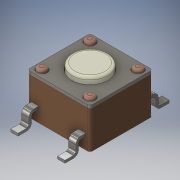
# Autodesk Inventor part: FSM2JSMAA
Saved by Autodesk Inventor 2016 (Build 200138000, 138)
## iProperties
Created: 2016-07-01
Part Number: FSM2JSMAA
Material: Generic
Document SubType Name: Modeling
Designer: Jonathan
Density: 1 g/cm^3
Appearance: Default
Author: Jonathan
Autodesk Inventor part; units mm, degrees
ref_plane "YZ Plane" through (0, 0, 0) normal (1, 0, 0) x (0, 1, 0)
ref_plane "XZ Plane" through (0, 0, 0) normal (0, 1, 0) x (-1, 0, 0)
ref_plane "XY Plane" through (0, 0, 0) normal (0, 0, 1) x (1, 0, 0)
sketch "Sketch1" plane through (0, 0, 0) normal (0, 1, 0) x (-1, 0, 0)
  line L0 (3, 3) -> (-3, 3)
  line L1 (-3, 3) -> (-3, -3)
  line L2 (-3, -3) -> (3, -3)
  line L3 (3, -3) -> (3, 3)
  point P0 (0, 0)
  point P1 (3, 0)
  point P2 (0, -3)
  dimension "d0" = 6
  dimension "d1" = 6
  constraints: 8 end point, 2 midpoint, 2 parallel, 1 horizontal, 1 horizontal alignment, 1 perpendicular, 1 vertical alignment
  measures "d0" distance of L2.end L0.start
  measures "d1" distance of L1.end L2.end
extrude "Extrusion1" add sketch "Sketch1" along normal blind 3.57
ref_plane "Work Plane1" through (2.25, 0, 3) normal (1, 0, 0) x (0, 0, -1)
sketch "Sketch2" plane through (2.25, 0, 3) normal (1, 0, 0) x (0, 0, -1)
  line L0 (6.45, 1.4) -> (6, 1.4)
  line L1 (6, 1.4) -> (6, 1.15)
  line L2 (6, 1.15) -> (6.45, 1.15)
  line L3 (6.7, 0.9) -> (6.7, 0.4)
  line L4 (6.95, 0.9) -> (6.95, 0.4)
  line L5 (7.2, 0.15) -> (8, 0.15)
  line L6 (8, 0.15) -> (8, -0.1)
  line L7 (8, -0.1) -> (7.2, -0.1)
  arc A0 (6.7, 0.9) -> (6.45, 1.15) centre (6.45, 0.9) ccw
  arc A1 (6.95, 0.9) -> (6.45, 1.4) centre (6.45, 0.9) ccw
  arc A2 (6.95, 0.4) -> (7.2, 0.15) centre (7.2, 0.4) ccw
  arc A3 (6.7, 0.4) -> (7.2, -0.1) centre (7.2, 0.4) ccw
  line L8 (6, 0) -> (6, 3.57) projected
  line L9 (0, 0) -> (6, 0) projected
  point P0 (3, 0)
  dimension "d6" = 0.25
  dimension "d7" = 0.8
  dimension "d8" = 2
  dimension "d9" = 1.5
  dimension "d11" = 0.1
  dimension "d12" = 0.7
  constraints: 16 end point, 8 point on circle, 8 tangent, 4 centre point, 4 perpendicular, 2 concentric, 2 horizontal, 2 vertical, 1 collinear, 1 equal radius
  measures "d6" distance between parallel lines of L3 L4
  measures "d7" distance of L6.end L7.end
  measures "d8" distance between parallel lines of L1 L6
  measures "d9" distance between parallel lines of L0 L7
  measures "d11" distance between parallel lines of L9 L7
  measures "d12" distance between parallel lines of L8 L3
extrude "Extrusion2" add sketch "Sketch2" along normal mid plane 0.7 separate body
mirror "Mirror1" about plane through (0, 0, 0) normal (1, 0, 0) of "Extrusion2" bodies 2
mirror "Mirror2" about plane through (0, 0, 0) normal (0, 0, 1) of "Extrusion2", "Mirror1" bodies 2
sketch "Sketch3" plane through (0, 3.57, 0) normal (0, 1, 0) x (1, 0, 0)
  line L0 (-3, -3) -> (3, -3) projected
  line L1 (3, 3) -> (-3, 3) projected
  line L2 (-3, -3) -> (3, -3)
  line L3 (3, -3) -> (3, 3)
  line L4 (3, 3) -> (-3, 3)
  line L5 (-3, 3) -> (-3, -3)
  circle A0 centre (0, 0) radius 1.75
  circle A1 centre (-2.3, -2.3) radius 0.5
  circle A2 centre (-2.3, 2.3) radius 0.5
  circle A3 centre (2.3, 2.3) radius 0.5
  circle A4 centre (2.3, -2.3) radius 0.5
  line L6 (-3, 3) -> (-3, -3) projected
  line L7 (-3, -3) -> (-2.3, -2.3) construction
  line L8 (-3, 3) -> (-2.3, 2.3) construction
  line L9 (2.3, 2.3) -> (3, 3) construction
  line L10 (3, -3) -> (3, 3) projected
  line L11 (2.3, -2.3) -> (3, -3) construction
  line L12 (-2.3, -2.3) -> (2.3, -2.3) construction
  line L13 (2.3, 2.3) -> (-2.3, 2.3) construction
  line L14 (-2.3, -2.3) -> (-2.3, 2.3) construction
  line L15 (2.3, 2.3) -> (2.3, -2.3) construction
  dimension "d15" = 3.5
  dimension "d16" = 1
  dimension "d17" = 0.7
  constraints: 24 end point, 5 centre point, 5 perpendicular, 4 parallel, 3 equal radius, 2 horizontal, 2 horizontal alignment, 2 vertical alignment, 1 coincident, 1 point on line
  measures "d15" diameter of A0
  measures "d16" diameter of A1
  measures "d17" distance from line of L5 L7.end
extrude "Extrusion3" add sketch "Sketch3" along normal blind 0.3 separate body
sketch "Sketch4" plane through (0, 3.57, 0) normal (0, 1, 0) x (1, 0, 0)
  circle A0 centre (-2.3, -2.3) radius 0.45
  circle A1 centre (-2.3, 2.3) radius 0.45
  circle A2 centre (2.3, 2.3) radius 0.45
  circle A3 centre (2.3, -2.3) radius 0.45
  circle A4 centre (-2.3, -2.3) radius 0.5 projected
  circle A5 centre (-2.3, 2.3) radius 0.5 projected
  circle A6 centre (2.3, 2.3) radius 0.5 projected
  circle A7 centre (2.3, -2.3) radius 0.5 projected
  point P0 (0, 0)
  dimension "d25" = 0.9
  dimension "d26" = 0.9
  dimension "d27" = 0.9
  dimension "d28" = 0.9
  constraints: 4 centre point, 4 concentric
  measures "d25" diameter of A0
  measures "d26" diameter of A3
  measures "d27" diameter of A2
  measures "d28" diameter of A1
extrude "Extrusion4" add sketch "Sketch4" along normal blind 0.6 separate body contours A0 | A1 | A2 | A3
sketch "Sketch5" plane through (0, 3.57, 0) normal (0, 1, 0) x (1, 0, 0)
  circle A0 centre (0, 0) radius 1.7
  circle A1 centre (0, 0) radius 1.75 projected
  dimension "d24" = 3.4
  constraints: 1 centre point, 1 concentric
  measures "d24" diameter of A0
extrude "Extrusion5" add sketch "Sketch5" along normal blind 0.9 separate body contours A0
fillet "Fillet1" radius 0.25 4 edges at (1.85, 4.17, 2.3) (1.85, 4.17, -2.3) (-2.75, 4.17, -2.3) (-2.75, 4.17, 2.3)
fillet "Fillet2" radius 0.25 1 edges at (-1.7, 4.47, 0)
fillet "Fillet3" radius 0.25 8 edges at (3, 1.785, 3) (3, 1.785, -3) (-3, 1.785, -3) (-3, 1.785, 3) (3, 3.72, 3) (3, 3.72, -3) (-3, 3.72, -3) (-3, 3.72, 3)
body "Solid1"
body "Solid2"
body "Solid3"
body "Solid4"
body "Solid5"
